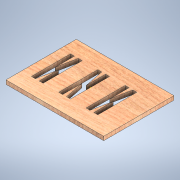
# Autodesk Inventor part: Parte A-B
Saved by Autodesk Inventor 2022 (Build 260153000, 153)
## iProperties
Created: 2023-02-12
Part Number: Parte A-B
Material: Madera (abedul)
Document SubType Name: Modeling
Designer: USUARIO
Density: 0.55 g/cm^3
Appearance: Abedul - Natural pulido
Author: USUARIO
Autodesk Inventor part; units mm, degrees
ref_plane "YZ Plane" through (0, 0, 0) normal (1, 0, 0) x (0, 1, 0)
ref_plane "XZ Plane" through (0, 0, 0) normal (0, 1, 0) x (-1, 0, 0)
ref_plane "XY Plane" through (0, 0, 0) normal (0, 0, 1) x (1, 0, 0)
sketch "Boceto1" plane through (0, 0, 0) normal (0, 1, 0) x (-1, 0, 0)
  point P0 (0, 0)
sketch "Boceto2" plane through (0, 0, 0) normal (0, 1, 0) x (-1, 0, 0)
  line L0 (125, 90) -> (-125, 90)
  line L1 (-125, 90) -> (-125, -90)
  line L2 (-125, -90) -> (125, -90)
  line L3 (125, -90) -> (125, 90)
  line L4 (125, 90) -> (-125, -90) construction
  line L5 (-125, 90) -> (125, -90) construction
  point P0 (0, 0)
  dimension "d0" = 250
  dimension "d1" = 180
  constraints: 12 end point, 2 midpoint, 2 parallel, 1 horizontal, 1 perpendicular
  measures "d0" distance of L2.end L1.end
  measures "d1" distance of L1.end L0.end
extrude "Extrusión1" add sketch "Boceto2" along normal blind 10
sketch "Boceto3" plane through (0, 10, 0) normal (0, 1, 0) x (1, 0, 0)
  point P0 (0, 0)
sketch "Boceto4" plane through (0, 10, 0) normal (0, 1, 0) x (1, 0, 0)
  line L0 (-125, 90) -> (-125, -90) projected
  line L1 (-125, 0) -> (-95, 0)
  line L2 (-125, 0) -> (-95, 0) construction
  line L3 (-100, -50) -> (-90, -50)
  line L4 (-90, -50) -> (-90, 50)
  line L5 (-90, 50) -> (-100, 50)
  line L6 (-100, 50) -> (-100, -50)
  line L7 (-100, -50) -> (-90, 50) construction
  line L8 (-90, -50) -> (-100, 50) construction
  line L9 (-90, -50) -> (-99.802, -48.0198)
  line L10 (-90, -50) -> (-80, -50) construction
  line L11 (-99.802, -48.0198) -> (-80, 50)
  line L12 (-90, -50) -> (-70.198, 48.0198)
  line L13 (-70.198, 48.0198) -> (-80, 50)
  line L14 (-90, 50) -> (-64.1181, 50)
  line L15 (-80, 50) -> (-70, 50)
  line L16 (-70, 50) -> (-70, -50)
  line L17 (-70, -50) -> (-80, -50)
  line L18 (-80, -50) -> (-80, 50)
  line L19 (-70, 0) -> (-50, 0)
  line L20 (-50, 0) -> (-50, -90)
  line L21 (0, -50) -> (-10, -50)
  line L22 (-10, -50) -> (-10, 50)
  line L23 (-10, 50) -> (0, 50)
  line L24 (0, 50) -> (0, -50)
  line L25 (0, -50) -> (-10, 50) construction
  line L26 (-10, -50) -> (0, 50) construction
  line L27 (-10, -50) -> (-0.198, -48.0198)
  line L28 (-10, -50) -> (-20, -50) construction
  line L29 (-0.198, -48.0198) -> (-20, 50)
  line L30 (-10, -50) -> (-29.802, 48.0198)
  line L31 (-29.802, 48.0198) -> (-20, 50)
  line L32 (-10, 50) -> (-35.8819, 50)
  line L33 (-20, 50) -> (-30, 50)
  line L34 (-30, 50) -> (-30, -50)
  line L35 (-30, -50) -> (-20, -50)
  line L36 (-20, -50) -> (-20, 50)
  line L37 (0, 0) -> (20, 0)
  line L38 (20, 0) -> (20, -90)
  line L39 (-125, -90) -> (125, -90) projected
  line L40 (50, -50) -> (69.802, 48.0198)
  line L41 (60, -50) -> (60, 50)
  line L42 (50, -50) -> (50, 50)
  line L43 (40, 50) -> (40, -50)
  line L44 (50, -50) -> (40, 50) construction
  line L45 (40, -50) -> (50, 50) construction
  line L46 (40.198, -48.0198) -> (60, 50)
  line L47 (50, 50) -> (40, 50)
  line L48 (50, 50) -> (75.8819, 50)
  line L49 (69.802, 48.0198) -> (60, 50)
  line L50 (60, 50) -> (70, 50)
  line L51 (70, -50) -> (60, -50)
  line L52 (50, -50) -> (60, -50) construction
  line L53 (50, -50) -> (40.198, -48.0198)
  line L54 (40, -50) -> (50, -50)
  line L55 (70, 50) -> (70, -50)
  point P0 (-5, 0)
  point P1 (-5, 0)
  point P2 (-30, 0)
  point P3 (40, 0)
  point P4 (45, 0)
  point P5 (45, 0)
  point P6 (70, 0)
  point P7 (50, 0.5)
  point P8 (60, -0.5)
  point P9 (-20, -0.5)
  point P10 (-10, 0.5)
  point P11 (-90, 0.5)
  point P12 (-80, -0.5)
  dimension "d4" = 30
  dimension "d5" = 0
  dimension "d6" = 10
  dimension "d7" = 100
  dimension "d8" = 10
  dimension "d10" = 100
  dimension "d11" = 100
  dimension "d12" = 10
  dimension "d13" = 100
  dimension "d14" = 20
  dimension "d15" = 20
  constraints: 108 end point, 31 symmetric about line, 8 horizontal, 8 midpoint, 6 perpendicular, 4 parallel, 4 point on line, 2 equal length
  measures "d4" distance of L1.start L1.end
  measures "d5" distance between parallel lines of L1 L2
  measures "d6" distance of L5.end L4.end
  measures "d7" distance of L4.end L3.end
  measures "d8" distance of L3.end L9.end
  measures "d10" distance of L9.end L11.end
  measures "d11" distance of L3.end L12.end
  measures "d12" distance of L16.end L17.end
  measures "d13" distance of L15.end L16.end
  measures "d14" distance of L19.start L19.end
  measures "d15" distance of L37.start L37.end
extrude "Extrusión2" cut sketch "Boceto4" against normal up to surface (10 mm away) contours L6 L5 L4 L11 L9 L3 | L9 L11 L4 | L4 L11 L18 L12 | L16 L17 L18 L12 L13 L14 | L13 L12 L18 | L21 L27 L29 L22 L23 L24 | L30 L36 L29 L22 | L22 L29 L27 | L36 L35 L34 L32 L31 L30 | L30 L31 L36 | L42 L46 L41 L40 | L53 L46 L42 | L54 L43 L47 L42 L46 L53 | L41 L49 L40 | L40 L49 L48 L55 L51 L41
equation "\"d0\" = alto_t"
equation "\"d1\" = ancho_t"
equation "\"d2\" = grueso_t"
equation "\"d4\" = d_ranura"
equation "\"d6\" = alto_p"
equation "\"d7\" = ancho_p"
equation "\"d8\" = alto_p"
equation "\"d10\" = ancho_p"
equation "\"d11\" = ancho_p"
equation "\"d12\" = alto_p"
equation "\"d13\" = ancho_p"
equation "\"d14\" = d_sim"
equation "\"d15\" = d_sim"
equation "\"ancho_t\" = 180"
equation "\"alto_t\" = 250"
equation "\"grueso_t\" = 10"
equation "\"d_ranura\" = 30"
equation "\"ancho_p\" = 100"
equation "\"alto_p\" = 10"
equation "\"angulo_p\" = 165deg"
equation "\"d_sim\" = 20"
